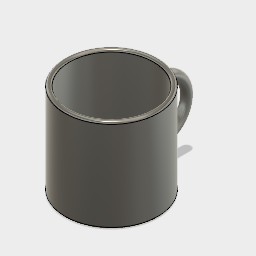
杯子 (Autodesk Fusion 360 design; units mm, degrees)
Autodesk Fusion 360 part; units mm, degrees
cylinder "圆柱体基本要素1" add diameter 100 height 100 placed x (1, 0, 0) y (0, 0, -1) z (0, 1, 0) at (0, 0, 0) makes body 1
cylinder "圆柱体基本要素2" add diameter 90 height 90 placed x (0, 0, -1) y (0, 1, 0) z (1, 0, 0) at (0, 35, 60) separate body makes body 2
torus "圆环体基本要素1" add centre line diameter 60 section diameter 10 placed x (0, 0, -1) y (0, 1, 0) z (1, 0, 0) at (0, 33.1481, -24.3739) separate body makes body 3
move_body "MoveFace1" bodies 3 to x (1, 0, 0) y (0, 1, 0) z (0, 0, 1) at (0, 17, -26) on bodies 3
combine "合并1" operation add target body 3 tool bodies 1
move_body "对齐1" bodies 2 to x (0, 1, 0) y (0, 0, 1) z (1, 0, 0) at (-60, 10, -35)
extrude "拉伸1" cut 1 faces at (-4.1569, 10, -25.5535) along direction (0, 1, 0) blind 2 on bodies 2 bodies 2
combine "合并2" operation cut target body 3 tool bodies 2
fillet "圆角1" radius 2.5 1 edges at (-46.6164, 100, 18.0808) on bodies 3
fillet "圆角2" radius 2 1 edges at (-46.6164, 0, -18.0808) on bodies 3
fillet "圆角3" radius 2.5 1 edges at (41.9547, 100, 16.2727) on bodies 3
sketch "草图9" plane through (0, 0, 0) normal (0, 1, 0) x (1, 0, 0)
  line L0 (16.5, 8.25) -> (-16.5, 8.25)
  line L1 (-16.5, 8.25) -> (-16.5, -8.25)
  line L2 (-16.5, -8.25) -> (16.5, -8.25)
  line L3 (16.5, -8.25) -> (16.5, 8.25)
  line L4 (16.5, 8.25) -> (-16.5, -8.25) construction
  line L5 (-16.5, 8.25) -> (16.5, -8.25) construction
  dimension "d12" = 16.5
  dimension "d13" = 33
  measures "d12" distance of L0.end L1.end
  measures "d13" distance of L1.end L2.end
extrude "拉伸2" cut sketch "草图9" along normal blind 10 bodies 3
